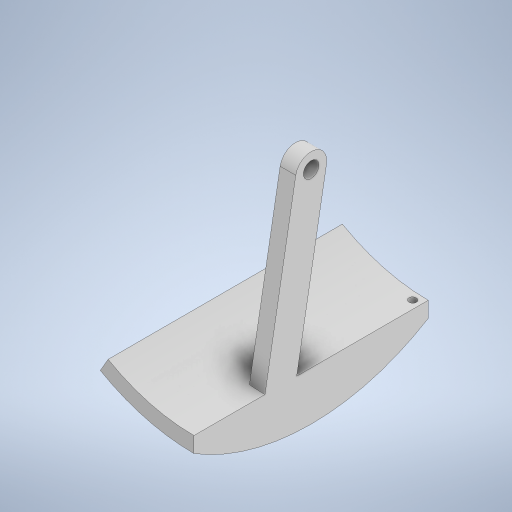
# Autodesk Inventor part: 受動歩行_ver4
Saved by Autodesk Inventor 2023 (Build 270158000, 158)
## iProperties
Created: 2024-06-12
Part Number: 受動歩行_ver4
Material: 一般
Document SubType Name: Modeling
Designer: babar
Density: 1 g/cm^3
Appearance: 既定
Author: babar
Autodesk Inventor part; units mm, degrees
ref_plane "YZ Plane" through (0, 0, 0) normal (1, 0, 0) x (0, 1, 0)
ref_plane "XZ Plane" through (0, 0, 0) normal (0, 1, 0) x (-1, 0, 0)
ref_plane "XY Plane" through (0, 0, 0) normal (0, 0, 1) x (1, 0, 0)
sketch "スケッチ1" plane through (0, 0, 0) normal (1, 0, 0) x (0, 1, 0)
  line L0 (-110, 75) -> (-110, -75)
  line L1 (-110, 0) -> (-125, 0)
  line L2 (-110, 75) -> (-120, 75)
  arc A0 (-120, 75) -> (-120, -75) centre (2.1096, 0) ccw
  line L3 (0, 75) -> (0, -75)
  line L4 (-110, -75) -> (-120, -75)
  point P0 (0, 0)
  dimension "d0" = 150
  dimension "d1" = 110
  dimension "d2" = 0
  dimension "d4" = 10
  constraints: 10 end point, 3 horizontal, 2 point on circle, 2 vertical, 1 centre point, 1 midpoint
  measures "d0" distance of L0.start L0.end
  measures "d1" distance from line of L0 point (0, 0)
  measures "d2" vertical distance of point (0, 0) L1.start
  measures "d4" distance of L0.start L2.end
revolve "回転1" add sketch "スケッチ1" angle 30 about axis through (0, 0, 75) along (0, 0, -1)
sketch "スケッチ2" plane through (0, -120, -75) normal (1, 0, 0) x (0, 0, -1)
  line L0 (-75, 120) -> (-95.8378, 1.8231) construction
  line L1 (-84.8481, 121.7365) -> (-105.6859, 3.5596)
  line L2 (-85.9897, 0.0866) -> (-65.1519, 118.2635)
  arc A0 (-65.1519, 118.2635) -> (-84.8481, 121.7365) centre (-75, 120) ccw
  arc A1 (-105.6859, 3.5596) -> (-85.9897, 0.0866) centre (-95.8378, 1.8231) ccw
  line L3 (-75, 120) -> (45, 120) construction
  point P0 (-85.4189, 60.9115)
  dimension "d6" = 120
  dimension "d7" = 100
  dimension "d8" = 20
  constraints: 10 end point, 4 point on circle, 4 tangent, 2 centre point, 1 equal length, 1 horizontal, 1 midpoint, 1 parallel
  measures "d6" distance of L0.start L0.end
  measures "d7" angle of L0 L3
  measures "d8" diameter of A1
extrude "押し出し1" add sketch "スケッチ2" against normal blind 10
sketch "スケッチ3" plane through (0, -120, 75) normal (1, 0, 0) x (0, 0, -1)
  point P0 (75, 120)
  point P1 (75, 120)
  constraints: 1 coincident
hole "穴1" at (0, 0, 0) direction (-1, 0, 0) diameter 10 end through all
sketch "スケッチ4" plane through (0, 0, 0) normal (0, 1, 0) x (-1, 0, 0)
  line L0 (0, -75) -> (55, -75) projected
  line L1 (0, -75) -> (0, 9.2417) projected
  point P0 (0, 0)
  point P1 (5, -70)
  dimension "d18" = 5
  dimension "d19" = 5
  measures "d18" distance from line of L0 point (5, -70)
  measures "d19" distance from line of L1 point (5, -70)
hole "穴2" at (-5, 0, -70) direction (0, -1, 0) diameter 4.8 end through all
sketch "スケッチ5" plane through (1.0548, 1.8269, 0) normal (-0.8660254, 0.5, 0) x (-0.5, -0.8660254, 0)
  ellipse E0 centre (7.1096, 0) end of major axis (7.1096, -5) minor radius 4.3301 projected
  line L0 (7.1096, 0) -> (183.6535, 22.8348)
  arc A0 (122.1096, -75) -> (122.1096, 75) centre (0, 0) ccw projected
  point P0 (2.1096, 0)
  point P1 (135, 16.5418)
  dimension "d27" = 135
  constraints: 2 end point, 1 point on line, 1 other
  measures "d27" horizontal distance of A0.centre point (135, 16.542)
hole "穴3" at (-66.4452, -115.0865, 16.5418) direction (0.8660254, -0.5, 0) diameter 4.8 depth 10
